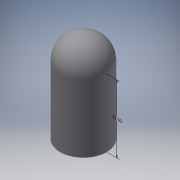
# Autodesk Inventor part: Dhgester
Saved by Autodesk Inventor 2019 (Build 230136000, 136)
## iProperties
Created: 2019-11-01
Part Number: Dhgester
Material: Generic
Document SubType Name: Modeling
Designer: Administrator
Density: 1 g/cm^3
Appearance: Default
Author: Administrator
Autodesk Inventor part; units mm, degrees
ref_plane "YZ Plane" through (0, 0, 0) normal (1, 0, 0) x (0, 1, 0)
ref_plane "XZ Plane" through (0, 0, 0) normal (0, 1, 0) x (-1, 0, 0)
ref_plane "XY Plane" through (0, 0, 0) normal (0, 0, 1) x (1, 0, 0)
sketch "Sketch1" plane through (0, 0, 0) normal (0, 1, 0) x (-1, 0, 0)
  circle A0 centre (0, 0) radius 285.75
  circle A1 centre (0, 0) radius 292.1
  dimension "d0" = 571.5
  dimension "d1" = 584.2
  constraints: 2 centre point, 2 coincident
  measures "d0" diameter of A0
  measures "d1" diameter of A1
extrude "Extrusion1" add sketch "Sketch1" along normal blind 850.9
sketch "Sketch2" plane through (0, 850.9, 0) normal (0, 1, 0) x (1, 0, 0)
  circle A0 centre (0, 0) radius 292.1 projected
  arc A1 (-292.1, 0) -> (292.1, 0) centre (0, 0) ccw
  circle A2 centre (0, 0) radius 285.75 projected
  line L0 (-292.1, 0) -> (292.1, 0)
  constraints: 4 point on circle, 2 end point, 1 centre point, 1 concentric, 1 horizontal
revolve "Revolution1" add sketch "Sketch2" angle 360 about axis through (-292.1, 850.9, 0) along (1, 0, 0) picked at (-284.3769, 55.6058) picked at (58.1784, 83.0313) contours L0 A2 A0 | L0 A2
body "Solid1"
